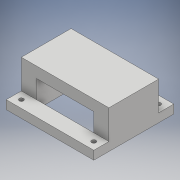
# Autodesk Inventor part: Sujetador para corte superior
Saved by Autodesk Inventor 2018 (Build 220112000, 112)
## iProperties
Created: 2019-05-21
Part Number: Sujetador para corte superior
Material: Generic
Document SubType Name: Modeling
Designer: Iván
Density: 1 g/cm^3
Appearance: Default
Author: Iván
Autodesk Inventor part; units mm, degrees
ref_plane "YZ Plane" through (0, 0, 0) normal (1, 0, 0) x (0, 1, 0)
ref_plane "XZ Plane" through (0, 0, 0) normal (0, 1, 0) x (-1, 0, 0)
ref_plane "XY Plane" through (0, 0, 0) normal (0, 0, 1) x (1, 0, 0)
sketch "Sketch1" plane through (0, 0, 0) normal (0, 0, 1) x (1, 0, 0)
  line L0 (-40.5, 37) -> (40.5, 37)
  line L1 (40.5, 37) -> (40.5, -37)
  line L2 (40.5, -37) -> (-40.5, -37)
  line L3 (-40.5, -37) -> (-40.5, 37)
  line L4 (-33.5, 30) -> (33.5, 30) construction
  line L5 (33.5, 30) -> (33.5, -30) construction
  line L6 (33.5, -30) -> (-33.5, -30) construction
  line L7 (-33.5, -30) -> (-33.5, 30) construction
  line L8 (26.5, 23) -> (-26.5, 23)
  line L9 (-26.5, 23) -> (-26.5, -23)
  line L10 (-26.5, -23) -> (26.5, -23)
  line L11 (26.5, -23) -> (26.5, 23)
  point P0 (0, 0)
  point P1 (0, 37)
  point P2 (-40.5, 0)
  point P3 (0, 30)
  point P4 (33.5, 0)
  dimension "d0" = 74
  dimension "d1" = 81
  dimension "d2" = 7
  dimension "d3" = 7
  dimension "d4" = 14
  constraints: 24 end point, 6 parallel, 4 coincident, 4 midpoint, 3 perpendicular, 2 horizontal, 2 horizontal alignment, 2 vertical alignment, 3 other
  measures "d0" distance of L0.end L1.end
  measures "d1" distance between parallel lines of L1 L3
  measures "d2" distance between parallel lines of L0 L4
  measures "d3" distance between parallel lines of L3 L7
  measures "d4" distance between parallel lines of L0 L8
extrude "Extrusion1" add sketch "Sketch1" along normal blind 8
hole "Hole1" at (-33.5, 30, 0) at (33.5, 30, 0) at (33.5, -30, 0) at (-33.5, -30, 0) direction (0, 0, 1) diameter 4 end through all
sketch "Sketch2" plane through (0, 0, 8) normal (0, 0, 1) x (1, 0, 0)
  line L0 (0, 0) -> (0, 37) construction
  line L1 (-26.5, 23) -> (-40.5, 23)
  line L2 (-40.5, 23) -> (-40.5, -23)
  line L3 (-40.5, -23) -> (-26.5, -23)
  line L4 (-26.5, -23) -> (-26.5, 23)
  line L5 (-26.5, 23) -> (26.5, 23) projected
  line L6 (-26.5, -23) -> (-26.5, 23) projected
  line L7 (-40.5, 37) -> (-40.5, -37) projected
  line L8 (26.5, -23) -> (-26.5, -23) projected
  line L9 (26.5, 23) -> (40.5, 23)
  line L10 (40.5, 23) -> (40.5, -23)
  line L11 (40.5, -23) -> (26.5, -23)
  line L12 (26.5, -23) -> (26.5, 23)
  line L13 (26.5, 23) -> (26.5, -23) projected
  line L14 (40.5, -37) -> (40.5, 37) projected
  constraints: 18 end point, 8 collinear, 4 parallel, 2 horizontal, 2 perpendicular, 1 vertical
extrude "Extrusion2" add sketch "Sketch2" along normal blind 27 contours L4 L3 L2 L1 | L9 L10 L11 L12
sketch "Sketch3" plane through (-26.5, -23, 0) normal (1, 0, 0) x (0, 0, -1)
  line L0 (-35, 0) -> (-25, 0)
  line L1 (-25, 0) -> (-25, 46)
  line L2 (-25, 46) -> (-35, 46)
  line L3 (-35, 46) -> (-35, 0)
  line L4 (-8, 46) -> (-35, 46) projected
  line L5 (-35, 0) -> (-35, 46) projected
  line L6 (-8, 0) -> (-35, 0) projected
  point P0 (0, 23)
  dimension "d16" = 10
  constraints: 8 end point, 3 collinear, 2 parallel, 1 horizontal, 1 perpendicular
  measures "d16" distance between parallel lines of L1 L3
extrude "Extrusion3" add sketch "Sketch3" along normal up to next
equation "\"d4\" = 2 * d2"
body "Solid1"
